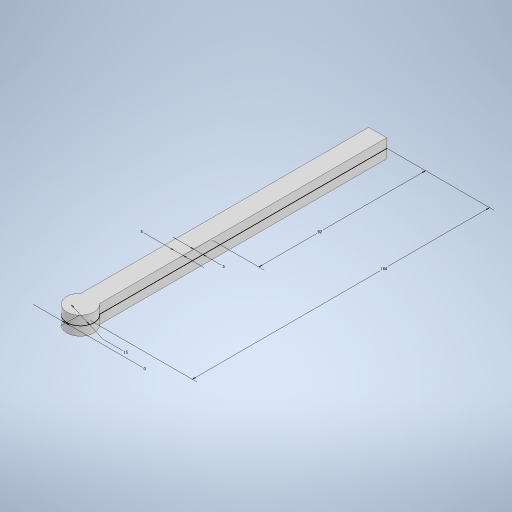
# Autodesk Inventor part: link_kp2heel
Saved by Autodesk Inventor 2024.3 (Build 283343000, 343)
## iProperties
Created: 2025-01-18
Part Number: link_kp2heel
Material: 一般
Document SubType Name: Modeling
Designer: yuu53
Density: 1 g/cm^3
Appearance: 既定
Author: yuu53
Autodesk Inventor part; units mm, degrees
ref_plane "YZ Plane" through (0, 0, 0) normal (1, 0, 0) x (0, 1, 0)
ref_plane "XZ Plane" through (0, 0, 0) normal (0, 1, 0) x (-1, 0, 0)
ref_plane "XY Plane" through (0, 0, 0) normal (0, 0, 1) x (1, 0, 0)
sketch "スケッチ1" plane through (0, 0, 0) normal (0, 1, 0) x (-1, 0, 0)
  line L0 (5, 72) -> (-5, 72)
  line L1 (-5, 72) -> (-5, -92)
  line L2 (-5, -92) -> (5, -92)
  line L3 (5, -92) -> (5, 72)
  circle A0 centre (0, 72) radius 7.5
  point P0 (0, 0)
  point P1 (-5, 66.4098)
  point P2 (5, 66.4098)
  point P3 (0, -92)
  dimension "d0" = 15
  dimension "d3" = 5
  dimension "d4" = 5
  dimension "d8" = 0
  dimension "d9" = 92
  dimension "d17" = 164
  constraints: 8 end point, 2 midpoint, 2 parallel, 1 centre point, 1 horizontal, 1 perpendicular
  measures "d0" diameter of A0
  measures "d3" distance from line of L1 point (0, 0)
  measures "d4" distance from line of L3 point (0, 0)
  measures "d8" distance of point (0, 72) A0.centre
  measures "d9" distance from line of point (0, 0) L2
  measures "d17" distance of L0.end L1.end
extrude "押し出し1" add sketch "スケッチ1" along normal blind 5 and the other way blind 5
